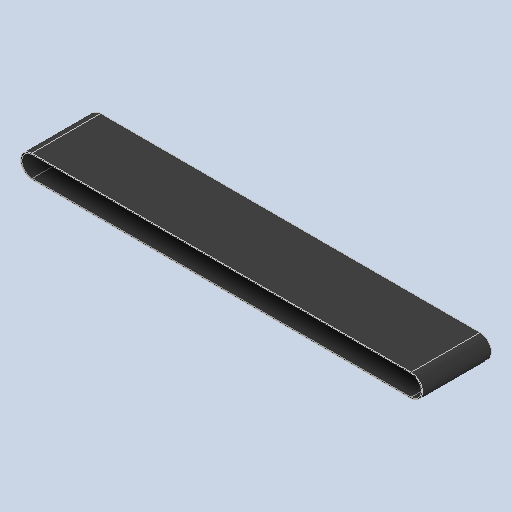
# Autodesk Inventor part: Banda
Saved by Autodesk Inventor 2025 (Build 290162000, 162)
## iProperties
Created: 2026-09-16
Part Number: Banda
Material: Caucho, Silicona
Document SubType Name: Modeling
Designer: ASUS
Density: 1.25 g/cm^3
Appearance: Caucho - Negro
Author: ASUS
Autodesk Inventor part; units mm, degrees
ref_plane "YZ Plane" through (0, 0, 0) normal (1, 0, 0) x (0, 1, 0)
ref_plane "XZ Plane" through (0, 0, 0) normal (0, 1, 0) x (-1, 0, 0)
ref_plane "XY Plane" through (0, 0, 0) normal (0, 0, 1) x (1, 0, 0)
sketch "Boceto1" plane through (0, 0, 0) normal (0, 0, 1) x (1, 0, 0)
  arc A0 (275.236, 12.4594) -> (275.236, 45.4594) centre (275.2631, 28.9594) ccw
  line L0 (275.236, 12.4594) -> (-274.7368, 12.4594)
  arc A1 (-274.7368, 45.4594) -> (-274.7368, 12.4594) centre (-274.7368, 28.9594) ccw
  line L1 (-274.7368, 45.4594) -> (275.236, 45.4594)
  point P0 (0, 0)
  point P1 (0, 43.9853)
  point P2 (0, 13.9594)
  point P3 (290.2632, 28.9594)
  point P4 (-289.7368, 28.9594)
  dimension "d5" = 580
  constraints: 4 end point, 4 point on circle, 2 centre point, 2 vertical alignment, 1 parallel
  measures "d5" distance of point (290.263, 28.959) point (-289.737, 28.959)
extrude "Extrusión1" add sketch "Boceto1" along normal blind 100
sketch "Boceto2" plane through (0, 0, 100) normal (0, 0, 1) x (1, 0, 0)
  line L0 (-274.4457, 43.9128) -> (274.9443, 43.9128)
  line L1 (275.236, 45.4594) -> (-274.7368, 45.4594) projected
  line L2 (274.9443, 13.9446) -> (-274.4457, 13.9446)
  line L3 (-274.7368, 12.4594) -> (275.236, 12.4594) projected
  arc A0 (-274.4457, 43.9128) -> (-274.4457, 13.9446) centre (-274.4457, 28.9287) ccw
  arc A1 (274.9443, 13.9446) -> (274.9443, 43.9128) centre (274.9443, 28.9287) ccw
  arc A2 (-274.7368, 45.4594) -> (-274.7368, 12.4594) centre (-274.7368, 28.9594) ccw projected
  point P0 (0, 0)
  dimension "d18" = 549.39
  constraints: 4 end point, 4 point on circle, 4 tangent, 2 centre point, 2 parallel
  measures "d18" distance of L0.start L0.end
extrude "Extrusión2" cut sketch "Boceto2" against normal blind 100
